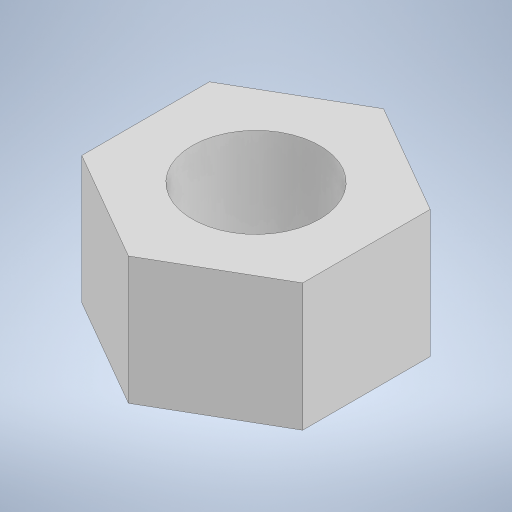
# Autodesk Inventor part: Part8
Saved by Autodesk Inventor 2024 (Build 280153000, 153)
## iProperties
Created: 2023-12-18
Part Number: Part8
Material: Generic
Document SubType Name: Modeling
Designer: SAHITYA
Density: 1 g/cm^3
Appearance: Default
Author: SAHITYA
Autodesk Inventor part; units mm, degrees
ref_plane "YZ Plane" through (0, 0, 0) normal (1, 0, 0) x (0, 1, 0)
ref_plane "XZ Plane" through (0, 0, 0) normal (0, 1, 0) x (-1, 0, 0)
ref_plane "XY Plane" through (0, 0, 0) normal (0, 0, 1) x (1, 0, 0)
sketch "Sketch1" plane through (0, 0, 0) normal (0, 1, 0) x (-1, 0, 0)
  circle A0 centre (0, 0) radius 1.5
  line L0 (0, -3) -> (-2.5981, -1.5)
  line L1 (-2.5981, -1.5) -> (-2.5981, 1.5)
  line L2 (-2.5981, 1.5) -> (0, 3)
  line L3 (0, 3) -> (2.5981, 1.5)
  line L4 (2.5981, 1.5) -> (2.5981, -1.5)
  line L5 (2.5981, -1.5) -> (0, -3)
  dimension "d0" = 3
  dimension "d1" = 3
  constraints: 12 end point, 2 coincident, 1 centre point, 13 other
  measures "d0" diameter of A0
  measures "d1" distance of L3.end L4.end
extrude "Extrusion1" add sketch "Sketch1" along normal blind 3
body "Solid1"
